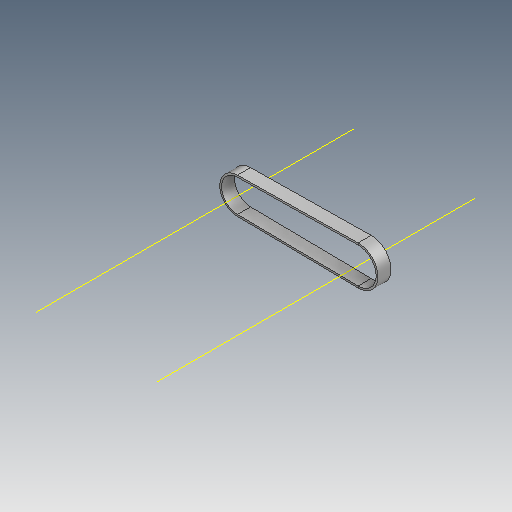
# Autodesk Inventor part: Synchronous Belt
Saved by Autodesk Inventor 2020.3 (Build 243373010, 373A)
## iProperties
CustomPartVersion: 1
Created: 2021-05-12
Part Number: Synchronous Belt
Material: Rubber
Document SubType Name: Modeling
Designer: marti
Density: 1 g/cm^3
Appearance: Rubber - Black - Version 1.1
Author: marti
Autodesk Inventor part; units mm, degrees
sketch "Sketch Path" plane through (0, 0, 0) normal (0, 0, 1) x (1, 0, 0)
  arc A0 (-0.2073, 15.1581) -> (-0.2073, -15.1581) centre (0, 0) ccw
  arc A1 (110.639, -16.6739) -> (110.639, 16.6739) centre (110.867, 0) ccw
  line L0 (110.639, -16.6739) -> (-0.2073, -15.1581)
  line L1 (-0.2073, 15.1581) -> (110.639, 16.6739)
  constraints: 4 end point, 4 point on circle, 2 centre point
ref_plane "Cross Section Plane" through (-0.2073, -15.1581, 0) normal (0.9999, -0.0137, 0) x (0, 0, 1)
ref_plane "Work Plane2" through (0, 0, 0) normal (0.309, 0.9511, 0) x (0, 0, 1)
ref_plane "Work Plane3" through (110.867, 0, 0) normal (-0.979, 0.2038, 0) x (0, 0, 1)
sketch "Cross Section" plane through (-0.2073, -15.1581, 0) normal (0.9999, -0.0137, 0) x (0, 0, 1)
  line L0 (-6, 1.27) -> (6, 1.27)
  line L1 (6, 1.27) -> (6, -0.381)
  line L2 (6, -0.381) -> (-6, -0.381)
  line L3 (-6, -0.381) -> (-6, 1.27)
  line L4 (-6, 0) -> (6, 0) construction
  point P0 (0, 0)
  point P1 (0, 0)
  dimension "d0" = 12
  dimension "d4" = 0.381
  dimension "d5" = 1.27
  constraints: 10 end point, 2 parallel, 2 point on line, 1 coincident, 1 horizontal, 1 midpoint, 1 perpendicular, 1 other
  measures "d0" distance between parallel lines of L1 L3
  measures "d4" distance between parallel lines of L2 L4
  measures "d5" distance between parallel lines of L4 L0
sweep "Belt" add profiles "Cross Section" path "Sketch Path"
equation "\"d4\" = da_a"
equation "\"d5\" = da_a2"
equation "\"da_B\" = 19.05"
equation "\"da_pb\" = 9.525"
equation "\"da_L\" = 321.76723"
equation "\"da_a\" = 0.381"
equation "\"da_S\" = 4.6482"
equation "\"da_Beta\" = 20deg"
equation "\"da_Ht\" = 1.905"
equation "\"da_H\" = 3.556"
equation "\"da_a2\" = 1.27"
body "Solid1"
